Autodesk Fusion 360 part; units mm, degrees
(part 4 of 8)
  spline S46 degree 5 poles (-31.9025, -58.9172) (-31.888, -58.9061) (-31.859, -58.884) (-31.8155, -58.8507) (-31.7578, -58.8063) (-31.6858, -58.7505) (-31.6141, -58.6945) (-31.5426, -58.6384) (-31.4714, -58.582) (-31.4004, -58.5254) (-31.3297, -58.4686) (-31.2593, -58.4117) (-31.1891, -58.3545) (-31.1191, -58.2971) (-31.0494, -58.2395) (-30.98, -58.1817) (-30.9109, -58.1237) (-30.842, -58.0655) (-30.7734, -58.0071) (-30.705, -57.9485) (-30.637, -57.8897) (-30.5692, -57.8306) (-30.5017, -57.7714) (-30.4345, -57.7119) (-30.3675, -57.6522) (-30.3009, -57.5923) (-30.2346, -57.5322) (-30.1685, -57.4719) (-30.1028, -57.4113) (-30.0373, -57.3505) (-29.9722, -57.2895) (-29.9073, -57.2283) (-29.8428, -57.1669) (-29.7786, -57.1052) (-29.7147, -57.0433) (-29.6512, -56.9812) (-29.588, -56.9188) (-29.5251, -56.8563) (-29.4626, -56.7934) (-29.4004, -56.7304) (-29.3385, -56.6671) (-29.277, -56.6035) (-29.2159, -56.5397) (-29.1551, -56.4757) (-29.0947, -56.4114) (-29.0347, -56.3469) (-28.9751, -56.2821) (-28.9158, -56.217) (-28.857, -56.1517) (-28.7986, -56.0861) (-28.7406, -56.0202) (-28.683, -55.9541) (-28.6369, -55.9004) (-28.6023, -55.8599) (-28.5792, -55.8327) (-28.5675, -55.8188) (-28.567, -55.8182) knots -1 -1 -1 -1 -1 -1 -0.985714 -0.971429 -0.957143 -0.942857 -0.928571 -0.914286 -0.9 -0.885714 -0.871429 -0.857143 -0.842857 -0.828571 -0.814286 -0.8 -0.785714 -0.771429 -0.757143 -0.742857 -0.728571 -0.714286 -0.7 -0.685714 -0.671429 -0.657143 -0.642857 -0.628571 -0.614286 -0.6 -0.585714 -0.571429 -0.557143 -0.542857 -0.528571 -0.514286 -0.5 -0.485714 -0.471429 -0.457143 -0.442857 -0.428571 -0.414286 -0.4 -0.385714 -0.371429 -0.357143 -0.342857 -0.328571 -0.314286 -0.3 -0.285714 -0.271429 -0.270845 -0.270845 -0.270845 -0.270845 -0.270845 -0.270845
  spline S47 degree 3 poles (-28.3236, -55.7689) (-28.3469, -55.7571) (-28.3722, -55.75) (-28.4241, -55.7458) (-28.4502, -55.7488) (-28.4928, -55.7624) (-28.5098, -55.7706) (-28.5409, -55.7914) (-28.5549, -55.8039) (-28.567, -55.8182) knots 0 0 0 0 0.007813 0.007813 0.015626 0.015626 0.021241 0.021241 0.026855 0.026855 0.026855 0.026855
  arc A24 (-28.3236, -55.7689) -> (-27.1157, -56.3661) centre (0, 0) ccw
  spline S48 degree 3 poles (-27.0071, -56.5894) (-27.0015, -56.564) (-27.0009, -56.5377) (-27.0098, -56.4864) (-27.0193, -56.4619) (-27.0431, -56.424) (-27.0553, -56.4096) (-27.0832, -56.3847) (-27.0988, -56.3743) (-27.1157, -56.3661) knots 0 0 0 0 0.007813 0.007813 0.015626 0.015626 0.021241 0.021241 0.026855 0.026855 0.026855 0.026855
  spline S49 degree 5 poles (-27.0071, -56.5894) (-27.0072, -56.5901) (-27.0112, -56.6079) (-27.0188, -56.6428) (-27.03, -56.6949) (-27.0446, -56.7641) (-27.0622, -56.85) (-27.0793, -56.9361) (-27.096, -57.0223) (-27.1122, -57.1087) (-27.1279, -57.1953) (-27.1432, -57.282) (-27.158, -57.3689) (-27.1724, -57.4559) (-27.1864, -57.5431) (-27.2, -57.6304) (-27.2131, -57.7178) (-27.2259, -57.8054) (-27.2382, -57.8931) (-27.2502, -57.981) (-27.2617, -58.0689) (-27.2729, -58.157) (-27.2837, -58.2452) (-27.2941, -58.3336) (-27.3041, -58.422) (-27.3137, -58.5106) (-27.323, -58.5993) (-27.3319, -58.6881) (-27.3405, -58.777) (-27.3487, -58.866) (-27.3565, -58.9551) (-27.364, -59.0443) (-27.3711, -59.1336) (-27.3779, -59.223) (-27.3843, -59.3126) (-27.3904, -59.4022) (-27.3962, -59.4919) (-27.4016, -59.5817) (-27.4067, -59.6716) (-27.4115, -59.7616) (-27.4159, -59.8516) (-27.42, -59.9418) (-27.4238, -60.032) (-27.4272, -60.1224) (-27.4303, -60.2128) (-27.4331, -60.3033) (-27.4356, -60.3939) (-27.4378, -60.4845) (-27.4397, -60.5753) (-27.4412, -60.6661) (-27.4425, -60.757) (-27.4434, -60.8479) (-27.444, -60.939) (-27.4443, -61.0119) (-27.4443, -61.0666) (-27.4443, -61.103) (-27.4443, -61.1213) knots 0.270845 0.270845 0.270845 0.270845 0.270845 0.270845 0.271429 0.285714 0.3 0.314286 0.328571 0.342857 0.357143 0.371429 0.385714 0.4 0.414286 0.428571 0.442857 0.457143 0.471429 0.485714 0.5 0.514286 0.528571 0.542857 0.557143 0.571429 0.585714 0.6 0.614286 0.628571 0.642857 0.657143 0.671429 0.685714 0.7 0.714286 0.728571 0.742857 0.757143 0.771429 0.785714 0.8 0.814286 0.828571 0.842857 0.857143 0.871429 0.885714 0.9 0.914286 0.928571 0.942857 0.957143 0.971429 0.985714 1 1 1 1 1 1
  arc A25 (-27.4443, -61.1213) -> (-26.0672, -61.7211) centre (0, 0) ccw
  spline S50 degree 5 poles (-26.0672, -61.7211) (-26.0538, -61.7087) (-26.0271, -61.6839) (-25.9871, -61.6466) (-25.9339, -61.5968) (-25.8676, -61.5343) (-25.8017, -61.4717) (-25.736, -61.4089) (-25.6705, -61.3459) (-25.6053, -61.2828) (-25.5404, -61.2194) (-25.4758, -61.1559) (-25.4114, -61.0922) (-25.3474, -61.0284) (-25.2836, -60.9643) (-25.2201, -60.9001) (-25.1568, -60.8357) (-25.0939, -60.7711) (-25.0312, -60.7064) (-24.9689, -60.6414) (-24.9068, -60.5763) (-24.845, -60.511) (-24.7836, -60.4455) (-24.7224, -60.3798) (-24.6615, -60.314) (-24.601, -60.2479) (-24.5408, -60.1817) (-24.4808, -60.1152) (-24.4212, -60.0486) (-24.362, -59.9818) (-24.303, -59.9148) (-24.2444, -59.8476) (-24.1861, -59.7803) (-24.1282, -59.7127) (-24.0706, -59.6449) (-24.0133, -59.5769) (-23.9564, -59.5088) (-23.8998, -59.4404) (-23.8437, -59.3718) (-23.7878, -59.3031) (-23.7324, -59.2341) (-23.6773, -59.1649) (-23.6226, -59.0955) (-23.5683, -59.0259) (-23.5144, -58.9561) (-23.4609, -58.8861) (-23.4078, -58.8158) (-23.3551, -58.7453) (-23.3029, -58.6747) (-23.2511, -58.6037) (-23.1997, -58.5326) (-23.1488, -58.4612) (-23.108, -58.4033) (-23.0775, -58.3597) (-23.0572, -58.3303) (-23.0468, -58.3153) (-23.0464, -58.3147) knots -1 -1 -1 -1 -1 -1 -0.985714 -0.971429 -0.957143 -0.942857 -0.928571 -0.914286 -0.9 -0.885714 -0.871429 -0.857143 -0.842857 -0.828571 -0.814286 -0.8 -0.785714 -0.771429 -0.757143 -0.742857 -0.728571 -0.714286 -0.7 -0.685714 -0.671429 -0.657143 -0.642857 -0.628571 -0.614286 -0.6 -0.585714 -0.571429 -0.557143 -0.542857 -0.528571 -0.514286 -0.5 -0.485714 -0.471429 -0.457143 -0.442857 -0.428571 -0.414286 -0.4 -0.385714 -0.371429 -0.357143 -0.342857 -0.328571 -0.314286 -0.3 -0.285714 -0.271429 -0.270845 -0.270845 -0.270845 -0.270845 -0.270845 -0.270845
  spline S51 degree 3 poles (-22.8089, -58.2422) (-22.8332, -58.2327) (-22.8591, -58.228) (-22.9111, -58.2289) (-22.9368, -58.2344) (-22.978, -58.252) (-22.994, -58.2618) (-23.023, -58.2855) (-23.0358, -58.2993) (-23.0464, -58.3147) knots 0 0 0 0 0.007813 0.007813 0.015626 0.015626 0.021241 0.021241 0.026855 0.026855 0.026855 0.026855
  arc A26 (-22.8089, -58.2422) -> (-21.549, -58.72) centre (0, 0) ccw
  spline S52 degree 3 poles (-21.4193, -58.9318) (-21.4162, -58.9059) (-21.4182, -58.8797) (-21.432, -58.8295) (-21.4438, -58.806) (-21.4712, -58.7706) (-21.4846, -58.7575) (-21.5148, -58.7354) (-21.5314, -58.7265) (-21.549, -58.72) knots 0 0 0 0 0.007813 0.007813 0.015626 0.015626 0.021241 0.021241 0.026855 0.026855 0.026855 0.026855
  spline S53 degree 5 poles (-21.4193, -58.9318) (-21.4194, -58.9325) (-21.4216, -58.9506) (-21.4258, -58.9861) (-21.432, -59.039) (-21.4398, -59.1093) (-21.449, -59.1965) (-21.4578, -59.2838) (-21.466, -59.3713) (-21.4738, -59.4588) (-21.4811, -59.5465) (-21.488, -59.6343) (-21.4943, -59.7222) (-21.5003, -59.8102) (-21.5058, -59.8983) (-21.5109, -59.9865) (-21.5155, -60.0748) (-21.5198, -60.1632) (-21.5236, -60.2517) (-21.527, -60.3403) (-21.53, -60.429) (-21.5326, -60.5177) (-21.5348, -60.6066) (-21.5366, -60.6955) (-21.5381, -60.7845) (-21.5391, -60.8736) (-21.5398, -60.9628) (-21.5401, -61.052) (-21.54, -61.1413) (-21.5396, -61.2307) (-21.5388, -61.3202) (-21.5376, -61.4097) (-21.5361, -61.4993) (-21.5342, -61.5889) (-21.532, -61.6786) (-21.5294, -61.7684) (-21.5265, -61.8583) (-21.5232, -61.9482) (-21.5196, -62.0381) (-21.5157, -62.1282) (-21.5114, -62.2182) (-21.5068, -62.3084) (-21.5018, -62.3986) (-21.4965, -62.4888) (-21.4909, -62.5791) (-21.485, -62.6695) (-21.4787, -62.7599) (-21.4721, -62.8503) (-21.4652, -62.9408) (-21.458, -63.0313) (-21.4505, -63.1219) (-21.4426, -63.2125) (-21.4344, -63.3032) (-21.4277, -63.3758) (-21.4224, -63.4302) (-21.4189, -63.4665) (-21.4171, -63.4847) knots 0.270845 0.270845 0.270845 0.270845 0.270845 0.270845 0.271429 0.285714 0.3 0.314286 0.328571 0.342857 0.357143 0.371429 0.385714 0.4 0.414286 0.428571 0.442857 0.457143 0.471429 0.485714 0.5 0.514286 0.528571 0.542857 0.557143 0.571429 0.585714 0.6 0.614286 0.628571 0.642857 0.657143 0.671429 0.685714 0.7 0.714286 0.728571 0.742857 0.757143 0.771429 0.785714 0.8 0.814286 0.828571 0.842857 0.857143 0.871429 0.885714 0.9 0.914286 0.928571 0.942857 0.957143 0.971429 0.985714 1 1 1 1 1 1
  arc A27 (-21.4171, -63.4847) -> (-19.9886, -63.9489) centre (0, 0) ccw
  spline S54 degree 5 poles (-19.9886, -63.9489) (-19.9765, -63.9352) (-19.9522, -63.9079) (-19.916, -63.867) (-19.8679, -63.8122) (-19.808, -63.7437) (-19.7483, -63.675) (-19.689, -63.6061) (-19.6299, -63.5371) (-19.5712, -63.468) (-19.5127, -63.3987) (-19.4545, -63.3292) (-19.3966, -63.2596) (-19.3389, -63.1899) (-19.2816, -63.12) (-19.2246, -63.0499) (-19.1679, -62.9797) (-19.1115, -62.9093) (-19.0554, -62.8388) (-18.9996, -62.7682) (-18.9441, -62.6974) (-18.8889, -62.6264) (-18.834, -62.5553) (-18.7795, -62.484) (-18.7253, -62.4126) (-18.6714, -62.341) (-18.6178, -62.2692) (-18.5646, -62.1973) (-18.5117, -62.1253) (-18.4591, -62.0531) (-18.4069, -61.9807) (-18.3551, -61.9082) (-18.3036, -61.8355) (-18.2524, -61.7626) (-18.2016, -61.6896) (-18.1512, -61.6164) (-18.1011, -61.5431) (-18.0514, -61.4696) (-18.0021, -61.3959) (-17.9532, -61.3221) (-17.9047, -61.2481) (-17.8565, -61.1739) (-17.8088, -61.0995) (-17.7615, -61.025) (-17.7145, -60.9503) (-17.6681, -60.8755) (-17.622, -60.8004) (-17.5764, -60.7252) (-17.5312, -60.6498) (-17.4865, -60.5742) (-17.4422, -60.4984) (-17.3984, -60.4225) (-17.3634, -60.3609) (-17.3373, -60.3145) (-17.3198, -60.2833) (-17.311, -60.2674) (-17.3106, -60.2668) knots -1 -1 -1 -1 -1 -1 -0.985714 -0.971429 -0.957143 -0.942857 -0.928571 -0.914286 -0.9 -0.885714 -0.871429 -0.857143 -0.842857 -0.828571 -0.814286 -0.8 -0.785714 -0.771429 -0.757143 -0.742857 -0.728571 -0.714286 -0.7 -0.685714 -0.671429 -0.657143 -0.642857 -0.628571 -0.614286 -0.6 -0.585714 -0.571429 -0.557143 -0.542857 -0.528571 -0.514286 -0.5 -0.485714 -0.471429 -0.457143 -0.442857 -0.428571 -0.414286 -0.4 -0.385714 -0.371429 -0.357143 -0.342857 -0.328571 -0.314286 -0.3 -0.285714 -0.271429 -0.270845 -0.270845 -0.270845 -0.270845 -0.270845 -0.270845
  spline S55 degree 3 poles (-17.0813, -60.1717) (-17.1063, -60.1646) (-17.1325, -60.1624) (-17.1843, -60.1683) (-17.2093, -60.1763) (-17.2486, -60.1978) (-17.2636, -60.2091) (-17.2902, -60.2355) (-17.3015, -60.2505) (-17.3106, -60.2668) knots 0 0 0 0 0.007813 0.007813 0.015626 0.015626 0.021241 0.021241 0.026855 0.026855 0.026855 0.026855
  arc A28 (-17.0813, -60.1717) -> (-15.7811, -60.5257) centre (0, 0) ccw
  spline S56 degree 3 poles (-15.6316, -60.724) (-15.631, -60.6979) (-15.6355, -60.672) (-15.6541, -60.6234) (-15.6681, -60.6011) (-15.6988, -60.5685) (-15.7134, -60.5568) (-15.7456, -60.5377) (-15.763, -60.5304) (-15.7811, -60.5257) knots 0 0 0 0 0.007813 0.007813 0.015626 0.015626 0.021241 0.021241 0.026855 0.026855 0.026855 0.026855
  spline S57 degree 5 poles (-15.6316, -60.724) (-15.6316, -60.7247) (-15.6321, -60.7429) (-15.6328, -60.7786) (-15.6338, -60.8318) (-15.6349, -60.9026) (-15.6356, -60.9903) (-15.6359, -61.0781) (-15.6357, -61.1659) (-15.6349, -61.2538) (-15.6338, -61.3418) (-15.6321, -61.4298) (-15.63, -61.5179) (-15.6274, -61.6061) (-15.6244, -61.6943) (-15.6209, -61.7826) (-15.617, -61.8709) (-15.6127, -61.9593) (-15.608, -62.0478) (-15.6028, -62.1363) (-15.5973, -62.2248) (-15.5913, -62.3134) (-15.5849, -62.4021) (-15.5781, -62.4908) (-15.571, -62.5795) (-15.5634, -62.6683) (-15.5555, -62.7571) (-15.5472, -62.8459) (-15.5385, -62.9348) (-15.5294, -63.0237) (-15.52, -63.1127) (-15.5102, -63.2017) (-15.5, -63.2907) (-15.4895, -63.3798) (-15.4786, -63.4688) (-15.4674, -63.558) (-15.4558, -63.6471) (-15.4439, -63.7363) (-15.4316, -63.8255) (-15.419, -63.9147) (-15.406, -64.0039) (-15.3927, -64.0932) (-15.3791, -64.1825) (-15.3651, -64.2718) (-15.3508, -64.3611) (-15.3362, -64.4505) (-15.3212, -64.5399) (-15.306, -64.6292) (-15.2903, -64.7187) (-15.2744, -64.8081) (-15.2582, -64.8975) (-15.2416, -64.987) (-15.2247, -65.0764) (-15.211, -65.148) (-15.2005, -65.2017) (-15.1935, -65.2375) (-15.19, -65.2554) knots 0.270845 0.270845 0.270845 0.270845 0.270845 0.270845 0.271429 0.285714 0.3 0.314286 0.328571 0.342857 0.357143 0.371429 0.385714 0.4 0.414286 0.428571 0.442857 0.457143 0.471429 0.485714 0.5 0.514286 0.528571 0.542857 0.557143 0.571429 0.585714 0.6 0.614286 0.628571 0.642857 0.657143 0.671429 0.685714 0.7 0.714286 0.728571 0.742857 0.757143 0.771429 0.785714 0.8 0.814286 0.828571 0.842857 0.857143 0.871429 0.885714 0.9 0.914286 0.928571 0.942857 0.957143 0.971429 0.985714 1 1 1 1 1 1
  arc A29 (-15.19, -65.2554) -> (-13.7233, -65.5795) centre (0, 0) ccw
  spline S58 degree 5 poles (-13.7233, -65.5795) (-13.7126, -65.5648) (-13.6911, -65.5353) (-13.659, -65.491) (-13.6163, -65.4319) (-13.5633, -65.3578) (-13.5106, -65.2837) (-13.4582, -65.2094) (-13.4061, -65.1351) (-13.3543, -65.0606) (-13.3027, -64.9859) (-13.2515, -64.9112) (-13.2006, -64.8363) (-13.15, -64.7613) (-13.0997, -64.6862) (-13.0497, -64.611) (-13, -64.5356) (-12.9506, -64.4602) (-12.9016, -64.3846) (-12.8529, -64.3089) (-12.8045, -64.233) (-12.7564, -64.1571) (-12.7087, -64.081) (-12.6612, -64.0048) (-12.6142, -63.9285) (-12.5674, -63.852) (-12.5211, -63.7754) (-12.475, -63.6987) (-12.4293, -63.6219) (-12.384, -63.545) (-12.339, -63.4679) (-12.2944, -63.3907) (-12.2501, -63.3134) (-12.2063, -63.2359) (-12.1627, -63.1583) (-12.1196, -63.0806) (-12.0769, -63.0028) (-12.0345, -62.9248) (-11.9925, -62.8468) (-11.951, -62.7685) (-11.9098, -62.6902) (-11.869, -62.6117) (-11.8287, -62.5331) (-11.7888, -62.4544) (-11.7493, -62.3755) (-11.7102, -62.2965) (-11.6716, -62.2174) (-11.6335, -62.1381) (-11.5958, -62.0587) (-11.5586, -61.9791) (-11.5218, -61.8994) (-11.4856, -61.8196) (-11.4567, -61.7549) (-11.4351, -61.7062) (-11.4208, -61.6735) (-11.4135, -61.6568) (-11.4132, -61.6562) knots -1 -1 -1 -1 -1 -1 -0.985714 -0.971429 -0.957143 -0.942857 -0.928571 -0.914286 -0.9 -0.885714 -0.871429 -0.857143 -0.842857 -0.828571 -0.814286 -0.8 -0.785714 -0.771429 -0.757143 -0.742857 -0.728571 -0.714286 -0.7 -0.685714 -0.671429 -0.657143 -0.642857 -0.628571 -0.614286 -0.6 -0.585714 -0.571429 -0.557143 -0.542857 -0.528571 -0.514286 -0.5 -0.485714 -0.471429 -0.457143 -0.442857 -0.428571 -0.414286 -0.4 -0.385714 -0.371429 -0.357143 -0.342857 -0.328571 -0.314286 -0.3 -0.285714 -0.271429 -0.270845 -0.270845 -0.270845 -0.270845 -0.270845 -0.270845
  spline S59 degree 3 poles (-11.1941, -61.5394) (-11.2197, -61.5347) (-11.246, -61.5351) (-11.297, -61.5459) (-11.3212, -61.5563) (-11.3581, -61.5815) (-11.372, -61.5942) (-11.3959, -61.623) (-11.4058, -61.639) (-11.4132, -61.6562) knots 0 0 0 0 0.007813 0.007813 0.015626 0.015626 0.021241 0.021241 0.026855 0.026855 0.026855 0.026855
  arc A30 (-11.1941, -61.5394) -> (-9.8659, -61.7662) centre (0, 0) ccw
  spline S60 degree 3 poles (-9.6979, -61.9491) (-9.6998, -61.9232) (-9.7068, -61.8978) (-9.73, -61.8512) (-9.7461, -61.8304) (-9.7798, -61.8009) (-9.7955, -61.7906) (-9.8294, -61.7747) (-9.8474, -61.7692) (-9.8659, -61.7662) knots 0 0 0 0 0.007813 0.007813 0.015626 0.015626 0.021241 0.021241 0.026855 0.026855 0.026855 0.026855
  spline S61 degree 5 poles (-9.6979, -61.9491) (-9.6979, -61.9499) (-9.6965, -61.968) (-9.6939, -62.0036) (-9.6897, -62.0567) (-9.6839, -62.1273) (-9.6762, -62.2146) (-9.668, -62.302) (-9.6593, -62.3894) (-9.6501, -62.4768) (-9.6404, -62.5643) (-9.6303, -62.6517) (-9.6197, -62.7392) (-9.6086, -62.8267) (-9.5971, -62.9143) (-9.5851, -63.0018) (-9.5727, -63.0894) (-9.5599, -63.1769) (-9.5466, -63.2645) (-9.533, -63.3521) (-9.5189, -63.4397) (-9.5044, -63.5273) (-9.4895, -63.6149) (-9.4742, -63.7025) (-9.4585, -63.7902) (-9.4424, -63.8778) (-9.426, -63.9654) (-9.4091, -64.053) (-9.3919, -64.1407) (-9.3743, -64.2283) (-9.3563, -64.3159) (-9.338, -64.4036) (-9.3193, -64.4912) (-9.3002, -64.5788) (-9.2808, -64.6665) (-9.261, -64.7541) (-9.2408, -64.8417) (-9.2204, -64.9293) (-9.1995, -65.0169) (-9.1784, -65.1045) (-9.1568, -65.192) (-9.135, -65.2796) (-9.1128, -65.3672) (-9.0903, -65.4547) (-9.0674, -65.5422) (-9.0442, -65.6298) (-9.0207, -65.7173) (-8.9969, -65.8048) (-8.9727, -65.8923) (-8.9482, -65.9797) (-8.9234, -66.0672) (-8.8983, -66.1546) (-8.8729, -66.242) (-8.8523, -66.3119) (-8.8367, -66.3644) (-8.8262, -66.3993) (-8.821, -66.4168) knots 0.270845 0.270845 0.270845 0.270845 0.270845 0.270845 0.271429 0.285714 0.3 0.314286 0.328571 0.342857 0.357143 0.371429 0.385714 0.4 0.414286 0.428571 0.442857 0.457143 0.471429 0.485714 0.5 0.514286 0.528571 0.542857 0.557143 0.571429 0.585714 0.6 0.614286 0.628571 0.642857 0.657143 0.671429 0.685714 0.7 0.714286 0.728571 0.742857 0.757143 0.771429 0.785714 0.8 0.814286 0.828571 0.842857 0.857143 0.871429 0.885714 0.9 0.914286 0.928571 0.942857 0.957143 0.971429 0.985714 1 1 1 1 1 1
  arc A31 (-8.821, -66.4168) -> (-7.3299, -66.5978) centre (0, 0) ccw
  spline S62 degree 5 poles (-7.3299, -66.5978) (-7.3206, -66.5821) (-7.3021, -66.5507) (-7.2744, -66.5035) (-7.2377, -66.4406) (-7.1921, -66.3618) (-7.1468, -66.2829) (-7.1018, -66.2039) (-7.0571, -66.1249) (-7.0127, -66.0457) (-6.9686, -65.9665) (-6.9248, -65.8871) (-6.8813, -65.8077) (-6.8382, -65.7282) (-6.7954, -65.6485) (-6.7529, -65.5688) (-6.7107, -65.4891) (-6.6689, -65.4092) (-6.6273, -65.3292) (-6.5862, -65.2491) (-6.5453, -65.169) (-6.5048, -65.0887) (-6.4646, -65.0084) (-6.4248, -64.928) (-6.3853, -64.8475) (-6.3462, -64.7668) (-6.3074, -64.6862) (-6.269, -64.6054) (-6.2309, -64.5245) (-6.1932, -64.4435) (-6.1559, -64.3625) (-6.1189, -64.2813) (-6.0823, -64.2001) (-6.0461, -64.1188) (-6.0103, -64.0374) (-5.9749, -63.9559) (-5.9398, -63.8743) (-5.9052, -63.7926) (-5.871, -63.7108) (-5.8371, -63.6289) (-5.8037, -63.547) (-5.7707, -63.465) (-5.7382, -63.3828) (-5.706, -63.3006) (-5.6743, -63.2183) (-5.6431, -63.1359) (-5.6123, -63.0534) (-5.582, -62.9708) (-5.5521, -62.8881) (-5.5228, -62.8053) (-5.4939, -62.7225) (-5.4655, -62.6395) (-5.443, -62.5724) (-5.4262, -62.5218) (-5.4151, -62.4879) (-5.4095, -62.4706) (-5.4093, -62.4699) knots -1 -1 -1 -1 -1 -1 -0.985714 -0.971429 -0.957143 -0.942857 -0.928571 -0.914286 -0.9 -0.885714 -0.871429 -0.857143 -0.842857 -0.828571 -0.814286 -0.8 -0.785714 -0.771429 -0.757143 -0.742857 -0.728571 -0.714286 -0.7 -0.685714 -0.671429 -0.657143 -0.642857 -0.628571 -0.614286 -0.6 -0.585714 -0.571429 -0.557143 -0.542857 -0.528571 -0.514286 -0.5 -0.485714 -0.471429 -0.457143 -0.442857 -0.428571 -0.414286 -0.4 -0.385714 -0.371429 -0.357143 -0.342857 -0.328571 -0.314286 -0.3 -0.285714 -0.271429 -0.270845 -0.270845 -0.270845 -0.270845 -0.270845 -0.270845
  spline S63 degree 3 poles (-5.2025, -62.3325) (-5.2284, -62.3303) (-5.2545, -62.3332) (-5.3042, -62.3489) (-5.3273, -62.3616) (-5.3616, -62.3902) (-5.3742, -62.4042) (-5.3952, -62.4352) (-5.4035, -62.4521) (-5.4093, -62.4699) knots 0 0 0 0 0.007813 0.007813 0.015626 0.015626 0.021241 0.021241 0.026855 0.026855 0.026855 0.026855
  arc A32 (-5.2025, -62.3325) -> (-3.8585, -62.4301) centre (0, 0) ccw
  spline S64 degree 3 poles (-3.6737, -62.5959) (-3.6781, -62.5703) (-3.6875, -62.5457) (-3.7151, -62.5015) (-3.7331, -62.4824) (-3.7695, -62.4563) (-3.7861, -62.4476) (-3.8214, -62.435) (-3.8398, -62.4312) (-3.8585, -62.4301) knots 0 0 0 0 0.007813 0.007813 0.015626 0.015626 0.021241 0.021241 0.026855 0.026855 0.026855 0.026855
  spline S65 degree 5 poles (-3.6737, -62.5959) (-3.6736, -62.5966) (-3.6705, -62.6146) (-3.6644, -62.6498) (-3.6552, -62.7022) (-3.6426, -62.7719) (-3.6265, -62.8581) (-3.6099, -62.9443) (-3.5928, -63.0304) (-3.5752, -63.1165) (-3.5571, -63.2026) (-3.5386, -63.2887) (-3.5196, -63.3748) (-3.5001, -63.4608) (-3.4802, -63.5468) (-3.4598, -63.6328) (-3.439, -63.7187) (-3.4178, -63.8047) (-3.3962, -63.8905) (-3.3741, -63.9764) (-3.3516, -64.0622) (-3.3287, -64.148) (-3.3055, -64.2338) (-3.2818, -64.3195) (-3.2577, -64.4052) (-3.2332, -64.4909) (-3.2084, -64.5765) (-3.1832, -64.6621) (-3.1576, -64.7477) (-3.1316, -64.8332) (-3.1052, -64.9187) (-3.0785, -65.0042) (-3.0515, -65.0896) (-3.024, -65.175) (-2.9962, -65.2603) (-2.9681, -65.3456) (-2.9396, -65.4308) (-2.9107, -65.5161) (-2.8816, -65.6012) (-2.852, -65.6864) (-2.8222, -65.7715) (-2.792, -65.8565) (-2.7614, -65.9415) (-2.7306, -66.0265) (-2.6994, -66.1114) (-2.6678, -66.1963) (-2.636, -66.2811) (-2.6038, -66.3659) (-2.5713, -66.4506) (-2.5385, -66.5353) (-2.5054, -66.62) (-2.4719, -66.7046) (-2.4382, -66.7891) (-2.4109, -66.8567) (-2.3904, -66.9074) (-2.3766, -66.9412) (-2.3697, -66.9581) knots 0.270845 0.270845 0.270845 0.270845 0.270845 0.270845 0.271429 0.285714 0.3 0.314286 0.328571 0.342857 0.357143 0.371429 0.385714 0.4 0.414286 0.428571 0.442857 0.457143 0.471429 0.485714 0.5 0.514286 0.528571 0.542857 0.557143 0.571429 0.585714 0.6 0.614286 0.628571 0.642857 0.657143 0.671429 0.685714 0.7 0.714286 0.728571 0.742857 0.757143 0.771429 0.785714 0.8 0.814286 0.828571 0.842857 0.857143 0.871429 0.885714 0.9 0.914286 0.928571 0.942857 0.957143 0.971429 0.985714 1 1 1 1 1 1
  arc A33 (-2.3697, -66.9581) -> (-0.8681, -66.9944) centre (0, 0) ccw
  spline S66 degree 5 poles (-0.8681, -66.9944) (-0.8604, -66.9778) (-0.845, -66.9448) (-0.822, -66.8951) (-0.7915, -66.8289) (-0.7537, -66.7461) (-0.7162, -66.6632) (-0.679, -66.5803) (-0.6421, -66.4973) (-0.6056, -66.4142) (-0.5694, -66.3311) (-0.5335, -66.2479) (-0.4979, -66.1646) (-0.4626, -66.0813) (-0.4277, -65.9979) (-0.3931, -65.9145) (-0.3588, -65.831) (-0.3248, -65.7475) (-0.2912, -65.6638) (-0.258, -65.5802) (-0.225, -65.4965) (-0.1925, -65.4127) (-0.1602, -65.3288) (-0.1283, -65.2449) (-0.0968, -65.161) (-0.0656, -65.077) (-0.0348, -64.9929) (-0.0044, -64.9088) (0.0257, -64.8246) (0.0554, -64.7404) (0.0847, -64.6561) (0.1137, -64.5718) (0.1423, -64.4874) (0.1705, -64.403) (0.1983, -64.3185) (0.2257, -64.2339) (0.2526, -64.1494) (0.2792, -64.0647) (0.3054, -63.98) (0.3312, -63.8953) (0.3565, -63.8105) (0.3815, -63.7256) (0.4059, -63.6407) (0.43, -63.5558) (0.4536, -63.4708) (0.4767, -63.3858) (0.4994, -63.3007) (0.5216, -63.2156) (0.5434, -63.1304) (0.5646, -63.0452) (0.5853, -62.9599) (0.6056, -62.8746) (0.6215, -62.8056) (0.6333, -62.7537) (0.6411, -62.7188) (0.645, -62.701) (0.6452, -62.7003) knots -1 -1 -1 -1 -1 -1 -0.985714 -0.971429 -0.957143 -0.942857 -0.928571 -0.914286 -0.9 -0.885714 -0.871429 -0.857143 -0.842857 -0.828571 -0.814286 -0.8 -0.785714 -0.771429 -0.757143 -0.742857 -0.728571 -0.714286 -0.7 -0.685714 -0.671429 -0.657143 -0.642857 -0.628571 -0.614286 -0.6 -0.585714 -0.571429 -0.557143 -0.542857 -0.528571 -0.514286 -0.5 -0.485714 -0.471429 -0.457143 -0.442857 -0.428571 -0.414286 -0.4 -0.385714 -0.371429 -0.357143 -0.342857 -0.328571 -0.314286 -0.3 -0.285714 -0.271429 -0.270845 -0.270845 -0.270845 -0.270845 -0.270845 -0.270845
  spline S67 degree 3 poles (0.8378, -62.5436) (0.8117, -62.5439) (0.786, -62.5494) (0.7381, -62.5698) (0.7164, -62.5846) (0.6849, -62.6164) (0.6737, -62.6315) (0.6558, -62.6644) (0.6492, -62.682) (0.6452, -62.7003) knots 0 0 0 0 0.007813 0.007813 0.015626 0.015626 0.021241 0.021241 0.026855 0.026855 0.026855 0.026855
  arc A34 (0.8378, -62.5436) -> (2.1849, -62.511) centre (0, 0) ccw
  spline S68 degree 3 poles (2.3848, -62.6583) (2.378, -62.6331) (2.3663, -62.6096) (2.3345, -62.5683) (2.3148, -62.551) (2.276, -62.5285) (2.2586, -62.5214) (2.2223, -62.5123) (2.2036, -62.5104) (2.1849, -62.511) knots 0 0 0 0 0.007813 0.007813 0.015626 0.015626 0.021241 0.021241 0.026855 0.026855 0.026855 0.026855
  spline S69 degree 5 poles (2.3848, -62.6583) (2.385, -62.659) (2.3898, -62.6765) (2.3993, -62.711) (2.4135, -62.7623) (2.4328, -62.8304) (2.4571, -62.9146) (2.482, -62.9988) (2.5073, -63.0829) (2.5331, -63.1669) (2.5594, -63.2509) (2.5862, -63.3348) (2.6134, -63.4186) (2.6411, -63.5024) (2.6692, -63.586) (2.6978, -63.6696) (2.7268, -63.7532) (2.7562, -63.8367) (2.786, -63.9201) (2.8163, -64.0034) (2.8469, -64.0866) (2.878, -64.1698) (2.9094, -64.253) (2.9413, -64.336) (2.9735, -64.419) (3.0061, -64.5019) (3.0391, -64.5847) (3.0725, -64.6675) (3.1062, -64.7502) (3.1403, -64.8328) (3.1748, -64.9153) (3.2097, -64.9978) (3.2448, -65.0802) (3.2804, -65.1626) (3.3163, -65.2448) (3.3525, -65.327) (3.3891, -65.4091) (3.4261, -65.4911) (3.4633, -65.5731) (3.5009, -65.655) (3.5389, -65.7368) (3.5771, -65.8185) (3.6157, -65.9002) (3.6547, -65.9818) (3.6939, -66.0633) (3.7335, -66.1447) (3.7734, -66.2261) (3.8136, -66.3074) (3.8541, -66.3886) (3.8949, -66.4697) (3.9361, -66.5508) (3.9775, -66.6318) (4.0193, -66.7127) (4.0529, -66.7773) (4.0783, -66.8258) (4.0953, -66.8581) (4.1038, -66.8742) knots 0.270845 0.270845 0.270845 0.270845 0.270845 0.270845 0.271429 0.285714 0.3 0.314286 0.328571 0.342857 0.357143 0.371429 0.385714 0.4 0.414286 0.428571 0.442857 0.457143 0.471429 0.485714 0.5 0.514286 0.528571 0.542857 0.557143 0.571429 0.585714 0.6 0.614286 0.628571 0.642857 0.657143 0.671429 0.685714 0.7 0.714286 0.728571 0.742857 0.757143 0.771429 0.785714 0.8 0.814286 0.828571 0.842857 0.857143 0.871429 0.885714 0.9 0.914286 0.928571 0.942857 0.957143 0.971429 0.985714 1 1 1 1 1 1
  arc A35 (4.1038, -66.8742) -> (5.6019, -66.7654) centre (0, 0) ccw
  spline S70 degree 5 poles (5.6019, -66.7654) (5.608, -66.7482) (5.6201, -66.7138) (5.6382, -66.6622) (5.6621, -66.5933) (5.6918, -66.5073) (5.7211, -66.4211) (5.7501, -66.335) (5.7788, -66.2488) (5.8071, -66.1626) (5.8352, -66.0764) (5.8629, -65.9901) (5.8903, -65.9038) (5.9173, -65.8175) (5.9441, -65.7311) (5.9704, -65.6447) (5.9965, -65.5583) (6.0222, -65.4719) (6.0476, -65.3854) (6.0726, -65.2989) (6.0973, -65.2124) (6.1217, -65.1259) (6.1457, -65.0393) (6.1693, -64.9527) (6.1926, -64.8661) (6.2155, -64.7795) (6.2381, -64.6929) (6.2602, -64.6062) (6.2821, -64.5195) (6.3035, -64.4328) (6.3246, -64.3461) (6.3452, -64.2594) (6.3655, -64.1726) (6.3854, -64.0859) (6.405, -63.9991) (6.4241, -63.9123) (6.4428, -63.8255) (6.4611, -63.7387) (6.479, -63.6519) (6.4964, -63.565) (6.5135, -63.4782) (6.5301, -63.3913) (6.5463, -63.3045) (6.562, -63.2176) (6.5773, -63.1307) (6.5921, -63.0438) (6.6065, -62.957) (6.6204, -62.8701) (6.6338, -62.7832) (6.6467, -62.6963) (6.6591, -62.6095) (6.671, -62.5226) (6.6803, -62.4524) (6.687, -62.3996) (6.6913, -62.3641) (6.6935, -62.346) (6.6936, -62.3453) knots -1 -1 -1 -1 -1 -1 -0.985714 -0.971429 -0.957143 -0.942857 -0.928571 -0.914286 -0.9 -0.885714 -0.871429 -0.857143 -0.842857 -0.828571 -0.814286 -0.8 -0.785714 -0.771429 -0.757143 -0.742857 -0.728571 -0.714286 -0.7 -0.685714 -0.671429 -0.657143 -0.642857 -0.628571 -0.614286 -0.6 -0.585714 -0.571429 -0.557143 -0.542857 -0.528571 -0.514286 -0.5 -0.485714 -0.471429 -0.457143 -0.442857 -0.428571 -0.414286 -0.4 -0.385714 -0.371429 -0.357143 -0.342857 -0.328571 -0.314286 -0.3 -0.285714 -0.271429 -0.270845 -0.270845 -0.270845 -0.270845 -0.270845 -0.270845
  spline S71 degree 3 poles (6.8702, -62.1708) (6.8443, -62.1736) (6.8192, -62.1815) (6.7735, -62.2065) (6.7533, -62.2233) (6.7251, -62.258) (6.7154, -62.2741) (6.7008, -62.3086) (6.6959, -62.3268) (6.6936, -62.3453) knots 0 0 0 0 0.007813 0.007813 0.015626 0.015626 0.021241 0.021241 0.026855 0.026855 0.026855 0.026855
  arc A36 (6.8702, -62.1708) -> (8.2079, -62.0083) centre (0, 0) ccw
  spline S72 degree 3 poles (8.4211, -62.1356) (8.4118, -62.1112) (8.3979, -62.0889) (8.3623, -62.0509) (8.341, -62.0356) (8.3003, -62.0169) (8.2823, -62.0116) (8.2452, -62.006) (8.2264, -62.0059) (8.2079, -62.0083) knots 0 0 0 0 0.007813 0.007813 0.015626 0.015626 0.021241 0.021241 0.026855 0.026855 0.026855 0.026855
  spline S73 degree 5 poles (8.4211, -62.1356) (8.4213, -62.1363) (8.4278, -62.1533) (8.4406, -62.1867) (8.4597, -62.2363) (8.4854, -62.3023) (8.5178, -62.3838) (8.5507, -62.4652) (8.584, -62.5464) (8.6178, -62.6276) (8.6521, -62.7086) (8.6868, -62.7895) (8.722, -62.8703) (8.7576, -62.951) (8.7937, -63.0316) (8.8302, -63.112) (8.8671, -63.1924) (8.9045, -63.2726) (8.9422, -63.3528) (8.9803, -63.4328) (9.0189, -63.5127) (9.0578, -63.5925) (9.0971, -63.6722) (9.1369, -63.7518) (9.177, -63.8313) (9.2174, -63.9106) (9.2583, -63.9899) (9.2995, -64.0691) (9.341, -64.1481) (9.3829, -64.227) (9.4252, -64.3059) (9.4679, -64.3846) (9.5108, -64.4632) (9.5542, -64.5417) (9.5978, -64.6202) (9.6418, -64.6985) (9.6862, -64.7766) (9.7309, -64.8547) (9.7759, -64.9327) (9.8212, -65.0106) (9.8669, -65.0884) (9.9129, -65.166) (9.9592, -65.2436) (10.0058, -65.321) (10.0527, -65.3984) (10.0999, -65.4756) (10.1475, -65.5527) (10.1954, -65.6298) (10.2435, -65.7067) (10.292, -65.7835) (10.3408, -65.8602) (10.3898, -65.9368) (10.4392, -66.0133) (10.4789, -66.0744) (10.5089, -66.1202) (10.5289, -66.1507) (10.5389, -66.1659) knots 0.270845 0.270845 0.270845 0.270845 0.270845 0.270845 0.271429 0.285714 0.3 0.314286 0.328571 0.342857 0.357143 0.371429 0.385714 0.4 0.414286 0.428571 0.442857 0.457143 0.471429 0.485714 0.5 0.514286 0.528571 0.542857 0.557143 0.571429 0.585714 0.6 0.614286 0.628571 0.642857 0.657143 0.671429 0.685714 0.7 0.714286 0.728571 0.742857 0.757143 0.771429 0.785714 0.8 0.814286 0.828571 0.842857 0.857143 0.871429 0.885714 0.9 0.914286 0.928571 0.942857 0.957143 0.971429 0.985714 1 1 1 1 1 1
  arc A37 (10.5389, -66.1659) -> (12.0195, -65.9131) centre (0, 0) ccw
  spline S74 degree 5 poles (12.0195, -65.9131) (12.0239, -65.8954) (12.0327, -65.8599) (12.0457, -65.8068) (12.0629, -65.736) (12.0841, -65.6474) (12.1049, -65.5589) (12.1255, -65.4703) (12.1457, -65.3818) (12.1656, -65.2933) (12.1852, -65.2047) (12.2045, -65.1162) (12.2234, -65.0276) (12.242, -64.9391) (12.2603, -64.8506) (12.2782, -64.762) (12.2958, -64.6735) (12.3131, -64.585) (12.33, -64.4965) (12.3466, -64.408) (12.3628, -64.3195) (12.3787, -64.231) (12.3942, -64.1426) (12.4093, -64.0541) (12.4242, -63.9657) (12.4386, -63.8772) (12.4527, -63.7888) (12.4664, -63.7004) (12.4798, -63.612) (12.4927, -63.5237) (12.5053, -63.4353) (12.5175, -63.347) (12.5294, -63.2587) (12.5408, -63.1704) (12.5519, -63.0822) (12.5625, -62.9939) (12.5727, -62.9057) (12.5826, -62.8175) (12.592, -62.7294) (12.601, -62.6413) (12.6096, -62.5532) (12.6177, -62.4651) (12.6255, -62.3771) (12.6327, -62.2891) (12.6396, -62.2012) (12.646, -62.1133) (12.6519, -62.0254) (12.6573, -61.9376) (12.6623, -61.8499) (12.6667, -61.7622) (12.6707, -61.6745) (12.6742, -61.5869) (12.6766, -61.5161) (12.6782, -61.4629) (12.6791, -61.4272) (12.6796, -61.409) (12.6796, -61.4083) knots -1 -1 -1 -1 -1 -1 -0.985714 -0.971429 -0.957143 -0.942857 -0.928571 -0.914286 -0.9 -0.885714 -0.871429 -0.857143 -0.842857 -0.828571 -0.814286 -0.8 -0.785714 -0.771429 -0.757143 -0.742857 -0.728571 -0.714286 -0.7 -0.685714 -0.671429 -0.657143 -0.642857 -0.628571 -0.614286 -0.6 -0.585714 -0.571429 -0.557143 -0.542857 -0.528571 -0.514286 -0.5 -0.485714 -0.471429 -0.457143 -0.442857 -0.428571 -0.414286 -0.4 -0.385714 -0.371429 -0.357143 -0.342857 -0.328571 -0.314286 -0.3 -0.285714 -0.271429 -0.270845 -0.270845 -0.270845 -0.270845 -0.270845 -0.270845
  spline S75 degree 3 poles (12.8385, -61.2175) (12.813, -61.2228) (12.7888, -61.2331) (12.7457, -61.2623) (12.7272, -61.281) (12.7025, -61.3183) (12.6944, -61.3353) (12.6831, -61.371) (12.68, -61.3895) (12.6796, -61.4083) knots 0 0 0 0 0.007813 0.007813 0.015626 0.015626 0.021241 0.021241 0.026855 0.026855 0.026855 0.026855
  arc A38 (12.8385, -61.2175) -> (14.1542, -60.9267) centre (0, 0) ccw
  spline S76 degree 3 poles (14.3787, -61.0328) (14.3672, -61.0094) (14.3512, -60.9886) (14.3121, -60.9542) (14.2893, -60.9409) (14.247, -60.9263) (14.2286, -60.9227) (14.1912, -60.9208) (14.1725, -60.9224) (14.1542, -60.9267) knots 0 0 0 0 0.007813 0.007813 0.015626 0.015626 0.021241 0.021241 0.026855 0.026855 0.026855 0.026855
  spline S77 degree 5 poles (14.3787, -61.0328) (14.379, -61.0334) (14.3871, -61.0497) (14.403, -61.0817) (14.4269, -61.1293) (14.4589, -61.1925) (14.4989, -61.2705) (14.5395, -61.3483) (14.5805, -61.426) (14.622, -61.5035) (14.6639, -61.5808) (14.7063, -61.658) (14.7491, -61.735) (14.7924, -61.8119) (14.8361, -61.8886) (14.8802, -61.9652) (14.9247, -62.0416) (14.9696, -62.1178) (15.0149, -62.194) (15.0606, -62.2699) (15.1066, -62.3458) (15.1531, -62.4214) (15.1999, -62.497) (15.2471, -62.5723) (15.2947, -62.6476) (15.3427, -62.7227) (15.3909, -62.7976) (15.4396, -62.8724) (15.4886, -62.9471) (15.5379, -63.0216) (15.5876, -63.096) (15.6377, -63.1703) (15.688, -63.2444) (15.7387, -63.3183) (15.7898, -63.3922) (15.8411, -63.4658) (15.8928, -63.5394) (15.9448, -63.6128) (15.9972, -63.6861) (16.0498, -63.7592) (16.1027, -63.8322) (16.156, -63.9051) (16.2096, -63.9778) (16.2634, -64.0504) (16.3176, -64.1228) (16.3721, -64.1952) (16.4269, -64.2673) (16.482, -64.3394) (16.5373, -64.4113) (16.593, -64.4831) (16.6489, -64.5547) (16.7052, -64.6262) (16.7617, -64.6976) (16.8071, -64.7546) (16.8413, -64.7973) (16.8642, -64.8257) (16.8756, -64.8399) knots 0.270845 0.270845 0.270845 0.270845 0.270845 0.270845 0.271429 0.285714 0.3 0.314286 0.328571 0.342857 0.357143 0.371429 0.385714 0.4 0.414286 0.428571 0.442857 0.457143 0.471429 0.485714 0.5 0.514286 0.528571 0.542857 0.557143 0.571429 0.585714 0.6 0.614286 0.628571 0.642857 0.657143 0.671429 0.685714 0.7 0.714286 0.728571 0.742857 0.757143 0.771429 0.785714 0.8 0.814286 0.828571 0.842857 0.857143 0.871429 0.885714 0.9 0.914286 0.928571 0.942857 0.957143 0.971429 0.985714 1 1 1 1 1 1
  arc A39 (16.8756, -64.8399) -> (18.3249, -64.4453) centre (0, 0) ccw
  spline S78 degree 5 poles (18.3249, -64.4453) (18.3276, -64.4273) (18.3329, -64.3912) (18.3407, -64.337) (18.351, -64.2649) (18.3636, -64.1747) (18.3758, -64.0845) (18.3877, -63.9944) (18.3993, -63.9043) (18.4105, -63.8143) (18.4215, -63.7243) (18.4321, -63.6343) (18.4424, -63.5443) (18.4524, -63.4544) (18.462, -63.3645) (18.4713, -63.2747) (18.4803, -63.1849) (18.4889, -63.0951) (18.4972, -63.0054) (18.5052, -62.9157) (18.5128, -62.8261) (18.5201, -62.7365) (18.527, -62.6469) (18.5335, -62.5574) (18.5397, -62.4679) (18.5456, -62.3785) (18.5511, -62.2892) (18.5562, -62.1998) (18.5609, -62.1106) (18.5653, -62.0214) (18.5693, -61.9322) (18.573, -61.8431) (18.5762, -61.7541) (18.5791, -61.6651) (18.5816, -61.5762) (18.5836, -61.4874) (18.5853, -61.3986) (18.5866, -61.3099) (18.5875, -61.2212) (18.5879, -61.1327) (18.588, -61.0442) (18.5876, -60.9557) (18.5868, -60.8674) (18.5855, -60.7791) (18.5839, -60.6909) (18.5817, -60.6028) (18.5791, -60.5148) (18.5761, -60.4269) (18.5725, -60.339) (18.5685, -60.2513) (18.564, -60.1637) (18.559, -60.0761) (18.5546, -60.0055) (18.551, -59.9523) (18.5485, -59.9167) (18.5472, -59.8985) (18.5471, -59.8978) knots -1 -1 -1 -1 -1 -1 -0.985714 -0.971429 -0.957143 -0.942857 -0.928571 -0.914286 -0.9 -0.885714 -0.871429 -0.857143 -0.842857 -0.828571 -0.814286 -0.8 -0.785714 -0.771429 -0.757143 -0.742857 -0.728571 -0.714286 -0.7 -0.685714 -0.671429 -0.657143 -0.642857 -0.628571 -0.614286 -0.6 -0.585714 -0.571429 -0.557143 -0.542857 -0.528571 -0.514286 -0.5 -0.485714 -0.471429 -0.457143 -0.442857 -0.428571 -0.414286 -0.4 -0.385714 -0.371429 -0.357143 -0.342857 -0.328571 -0.314286 -0.3 -0.285714 -0.271429 -0.270845 -0.270845 -0.270845 -0.270845 -0.270845 -0.270845
  spline S79 degree 3 poles (18.6869, -59.6926) (18.662, -59.7004) (18.6389, -59.7129) (18.5988, -59.7462) (18.5822, -59.7666) (18.5612, -59.8061) (18.5548, -59.8238) (18.5471, -59.8604) (18.5458, -59.8792) (18.5471, -59.8978) knots 0 0 0 0 0.007813 0.007813 0.015626 0.015626 0.021241 0.021241 0.026855 0.026855 0.026855 0.026855
  arc A40 (18.6869, -59.6926) -> (19.9684, -59.2762) centre (0, 0) ccw
  spline S80 degree 3 poles (20.2021, -59.3601) (20.1884, -59.338) (20.1704, -59.3188) (20.1282, -59.2883) (20.1043, -59.2773) (20.0608, -59.2669) (20.042, -59.2651) (20.0046, -59.2667) (19.9862, -59.2702) (19.9684, -59.2762) knots 0 0 0 0 0.007813 0.007813 0.015626 0.015626 0.021241 0.021241 0.026855 0.026855 0.026855 0.026855
  spline S81 degree 5 poles (20.2021, -59.3601) (20.2025, -59.3607) (20.2121, -59.3762) (20.231, -59.4065) (20.2594, -59.4516) (20.2973, -59.5113) (20.3447, -59.5851) (20.3926, -59.6586) (20.4409, -59.732) (20.4897, -59.8051) (20.5389, -59.878) (20.5885, -59.9508) (20.6386, -60.0233) (20.6891, -60.0957) (20.7399, -60.1678) (20.7912, -60.2397) (20.8429, -60.3115) (20.8949, -60.3831) (20.9474, -60.4545) (21.0002, -60.5257) (21.0533, -60.5967) (21.1069, -60.6675) (21.1608, -60.7382) (21.2151, -60.8087) (21.2697, -60.879) (21.3246, -60.9491) (21.3799, -61.019) (21.4356, -61.0888) (21.4916, -61.1584) (21.5479, -61.2278) (21.6045, -61.297) (21.6615, -61.3661) (21.7188, -61.435) (21.7764, -61.5037) (21.8343, -61.5723) (21.8925, -61.6407) (21.9511, -61.7089) (22.0099, -61.7769) (22.0691, -61.8448) (22.1285, -61.9125) (22.1883, -61.9801) (22.2483, -62.0475) (22.3086, -62.1147) (22.3693, -62.1817) (22.4302, -62.2486) (22.4914, -62.3153) (22.5529, -62.3819) (22.6147, -62.4483) (22.6767, -62.5145) (22.739, -62.5806) (22.8016, -62.6465) (22.8645, -62.7122) (22.9277, -62.7778) (22.9784, -62.8302) (23.0166, -62.8693) (23.0421, -62.8954) (23.0548, -62.9085) knots 0.270845 0.270845 0.270845 0.270845 0.270845 0.270845 0.271429 0.285714 0.3 0.314286 0.328571 0.342857 0.357143 0.371429 0.385714 0.4 0.414286 0.428571 0.442857 0.457143 0.471429 0.485714 0.5 0.514286 0.528571 0.542857 0.557143 0.571429 0.585714 0.6 0.614286 0.628571 0.642857 0.657143 0.671429 0.685714 0.7 0.714286 0.728571 0.742857 0.757143 0.771429 0.785714 0.8 0.814286 0.828571 0.842857 0.857143 0.871429 0.885714 0.9 0.914286 0.928571 0.942857 0.957143 0.971429 0.985714 1 1 1 1 1 1
  arc A41 (23.0548, -62.9085) -> (24.4592, -62.3758) centre (0, 0) ccw
  spline S82 degree 5 poles (24.4592, -62.3758) (24.4602, -62.3576) (24.4619, -62.3212) (24.4645, -62.2665) (24.4678, -62.1937) (24.4716, -62.1028) (24.475, -62.0119) (24.4782, -61.921) (24.481, -61.8302) (24.4836, -61.7395) (24.4858, -61.6489) (24.4877, -61.5583) (24.4892, -61.4677) (24.4905, -61.3773) (24.4914, -61.2869) (24.492, -61.1966) (24.4922, -61.1063) (24.4922, -61.0161) (24.4918, -60.926) (24.491, -60.836) (24.49, -60.746) (24.4885, -60.6561) (24.4868, -60.5663) (24.4847, -60.4766) (24.4822, -60.387) (24.4794, -60.2974) (24.4762, -60.2079) (24.4727, -60.1185) (24.4688, -60.0292) (24.4646, -59.94) (24.46, -59.8509) (24.455, -59.7619) (24.4496, -59.673) (24.4439, -59.5841) (24.4378, -59.4954) (24.4313, -59.4068) (24.4244, -59.3182) (24.4171, -59.2298) (24.4094, -59.1415) (24.4013, -59.0533) (24.3928, -58.9652) (24.3839, -58.8772) (24.3746, -58.7894) (24.3648, -58.7016) (24.3546, -58.614) (24.344, -58.5265) (24.3329, -58.4392) (24.3214, -58.3519) (24.3094, -58.2649) (24.2969, -58.1779) (24.284, -58.0911) (24.2706, -58.0045) (24.2593, -57.9346) (24.2506, -57.882) (24.2447, -57.8468) (24.2416, -57.8288) (24.2415, -57.8281) knots -1 -1 -1 -1 -1 -1 -0.985714 -0.971429 -0.957143 -0.942857 -0.928571 -0.914286 -0.9 -0.885714 -0.871429 -0.857143 -0.842857 -0.828571 -0.814286 -0.8 -0.785714 -0.771429 -0.757143 -0.742857 -0.728571 -0.714286 -0.7 -0.685714 -0.671429 -0.657143 -0.642857 -0.628571 -0.614286 -0.6 -0.585714 -0.571429 -0.557143 -0.542857 -0.528571 -0.514286 -0.5 -0.485714 -0.471429 -0.457143 -0.442857 -0.428571 -0.414286 -0.4 -0.385714 -0.371429 -0.357143 -0.342857 -0.328571 -0.314286 -0.3 -0.285714 -0.271429 -0.270845 -0.270845 -0.270845 -0.270845 -0.270845 -0.270845
  spline S83 degree 3 poles (24.3608, -57.6104) (24.3368, -57.6205) (24.315, -57.6352) (24.2784, -57.6722) (24.2638, -57.6941) (24.2467, -57.7355) (24.242, -57.7537) (24.2378, -57.7909) (24.2384, -57.8097) (24.2415, -57.8281) knots 0 0 0 0 0.007813 0.007813 0.015626 0.015626 0.021241 0.021241 0.026855 0.026855 0.026855 0.026855
  arc A42 (24.3608, -57.6104) -> (25.5962, -57.0722) centre (0, 0) ccw
  spline S84 degree 3 poles (25.8369, -57.1332) (25.8211, -57.1125) (25.8013, -57.0951) (25.7564, -57.0689) (25.7315, -57.0602) (25.6872, -57.054) (25.6684, -57.0541) (25.6313, -57.0593) (25.6133, -57.0646) (25.5962, -57.0722) knots 0 0 0 0 0.007813 0.007813 0.015626 0.015626 0.021241 0.021241 0.026855 0.026855 0.026855 0.026855
  spline S85 degree 5 poles (25.8369, -57.1332) (25.8373, -57.1338) (25.8484, -57.1482) (25.8701, -57.1766) (25.9027, -57.2187) (25.9462, -57.2745) (26.0005, -57.3434) (26.0553, -57.412) (26.1105, -57.4803) (26.166, -57.5484) (26.2221, -57.6162) (26.2785, -57.6838) (26.3353, -57.7512) (26.3925, -57.8183) (26.4501, -57.8852) (26.5081, -57.9519) (26.5665, -58.0183) (26.6252, -58.0845) (26.6843, -58.1505) (26.7437, -58.2163) (26.8035, -58.2819) (26.8636, -58.3472) (26.9241, -58.4123) (26.9849, -58.4772) (27.046, -58.5419) (27.1075, -58.6064) (27.1693, -58.6707) (27.2314, -58.7348) (27.2939, -58.7986) (27.3566, -58.8623) (27.4197, -58.9257) (27.483, -58.989) (27.5467, -59.052) (27.6107, -59.1149) (27.6749, -59.1775) (27.7395, -59.24) (27.8044, -59.3022) (27.8695, -59.3643) (27.9349, -59.4261) (28.0006, -59.4878) (28.0666, -59.5493) (28.1329, -59.6105) (28.1994, -59.6716) (28.2663, -59.7325) (28.3333, -59.7932) (28.4007, -59.8537) (28.4683, -59.914) (28.5362, -59.9741) (28.6044, -60.0341) (28.6728, -60.0938) (28.7414, -60.1534) (28.8104, -60.2127) (28.8796, -60.2719) (28.9351, -60.3191) (28.9769, -60.3544) (29.0048, -60.3779) (29.0187, -60.3897) knots 0.270845 0.270845 0.270845 0.270845 0.270845 0.270845 0.271429 0.285714 0.3 0.314286 0.328571 0.342857 0.357143 0.371429 0.385714 0.4 0.414286 0.428571 0.442857 0.457143 0.471429 0.485714 0.5 0.514286 0.528571 0.542857 0.557143 0.571429 0.585714 0.6 0.614286 0.628571 0.642857 0.657143 0.671429 0.685714 0.7 0.714286 0.728571 0.742857 0.757143 0.771429 0.785714 0.8 0.814286 0.828571 0.842857 0.857143 0.871429 0.885714 0.9 0.914286 0.928571 0.942857 0.957143 0.971429 0.985714 1 1 1 1 1 1
  arc A43 (29.0187, -60.3897) -> (30.3652, -59.724) centre (0, 0) ccw
  spline S86 degree 5 poles (30.3652, -59.724) (30.3643, -59.7058) (30.3626, -59.6693) (30.3599, -59.6147) (30.3561, -59.5419) (30.3511, -59.451) (30.3458, -59.3602) (30.3402, -59.2695) (30.3342, -59.1788) (30.328, -59.0883) (30.3214, -58.9978) (30.3146, -58.9075) (30.3074, -58.8172) (30.2999, -58.7271) (30.2921, -58.637) (30.284, -58.547) (30.2755, -58.4572) (30.2667, -58.3674) (30.2576, -58.2778) (30.2482, -58.1882) (30.2385, -58.0988) (30.2284, -58.0095) (30.218, -57.9203) (30.2072, -57.8312) (30.1961, -57.7422) (30.1847, -57.6533) (30.1729, -57.5646) (30.1607, -57.4759) (30.1483, -57.3874) (30.1354, -57.299) (30.1222, -57.2108) (30.1087, -57.1227) (30.0948, -57.0347) (30.0805, -56.9468) (30.0658, -56.8591) (30.0508, -56.7715) (30.0354, -56.684) (30.0196, -56.5967) (30.0034, -56.5096) (29.9869, -56.4225) (29.9699, -56.3357) (29.9525, -56.249) (29.9348, -56.1624) (29.9166, -56.076) (29.898, -55.9898) (29.879, -55.9038) (29.8595, -55.8179) (29.8396, -55.7322) (29.8193, -55.6467) (29.7985, -55.5613) (29.7772, -55.4762) (29.7555, -55.3912) (29.7376, -55.3227) (29.7238, -55.2713) (29.7145, -55.2368) (29.7098, -55.2192) (29.7096, -55.2185) knots -1 -1 -1 -1 -1 -1 -0.985714 -0.971429 -0.957143 -0.942857 -0.928571 -0.914286 -0.9 -0.885714 -0.871429 -0.857143 -0.842857 -0.828571 -0.814286 -0.8 -0.785714 -0.771429 -0.757143 -0.742857 -0.728571 -0.714286 -0.7 -0.685714 -0.671429 -0.657143 -0.642857 -0.628571 -0.614286 -0.6 -0.585714 -0.571429 -0.557143 -0.542857 -0.528571 -0.514286 -0.5 -0.485714 -0.471429 -0.457143 -0.442857 -0.428571 -0.414286 -0.4 -0.385714 -0.371429 -0.357143 -0.342857 -0.328571 -0.314286 -0.3 -0.285714 -0.271429 -0.270845 -0.270845 -0.270845 -0.270845 -0.270845 -0.270845
  spline S87 degree 3 poles (29.8073, -54.9903) (29.7844, -55.0027) (29.7641, -55.0194) (29.7312, -55.0598) (29.7188, -55.083) (29.7058, -55.1258) (29.7029, -55.1444) (29.7023, -55.1818) (29.7047, -55.2005) (29.7096, -55.2185) knots 0 0 0 0 0.007813 0.007813 0.015626 0.015626 0.021241 0.021241 0.026855 0.026855 0.026855 0.026855
  arc A44 (29.8073, -54.9903) -> (30.9849, -54.3354) centre (0, 0) ccw
  spline S88 degree 3 poles (31.2304, -54.3729) (31.2127, -54.3538) (31.1914, -54.3384) (31.1441, -54.3166) (31.1185, -54.3104) (31.0738, -54.3085) (31.0551, -54.3104) (31.0187, -54.3192) (31.0012, -54.3261) (30.9849, -54.3354) knots 0 0 0 0 0.007813 0.007813 0.015626 0.015626 0.021241 0.021241 0.026855 0.026855 0.026855 0.026855
  spline S89 degree 5 poles (31.2304, -54.3729) (31.2309, -54.3734) (31.2433, -54.3867) (31.2677, -54.4128) (31.3042, -54.4516) (31.3529, -54.503) (31.4136, -54.5663) (31.4747, -54.6292) (31.5362, -54.6919) (31.5981, -54.7543) (31.6604, -54.8165) (31.7231, -54.8783) (31.7862, -54.9399) (31.8496, -55.0012) (31.9134, -55.0622) (31.9775, -55.1229) (32.042, -55.1834) (32.1069, -55.2437) (32.172, -55.3037) (32.2375, -55.3634) (32.3034, -55.4229) (32.3695, -55.4821) (32.436, -55.5411) (32.5028, -55.5998) (32.5699, -55.6583) (32.6373, -55.7166) (32.705, -55.7746) (32.773, -55.8324) (32.8413, -55.8899) (32.9099, -55.9472) (32.9788, -56.0043) (33.048, -56.0611) (33.1175, -56.1177) (33.1872, -56.1741) (33.2572, -56.2302) (33.3275, -56.2862) (33.398, -56.3419) (33.4689, -56.3973) (33.54, -56.4526) (33.6113, -56.5076) (33.6829, -56.5624) (33.7548, -56.617) (33.8269, -56.6714) (33.8993, -56.7256) (33.9719, -56.7795) (34.0448, -56.8332) (34.118, -56.8867) (34.1913, -56.94) (34.265, -56.9931) (34.3388, -57.0459) (34.4129, -57.0986) (34.4872, -57.151) (34.5618, -57.2033) (34.6217, -57.2449) (34.6666, -57.276) (34.6967, -57.2967) (34.7117, -57.307) knots 0.270845 0.270845 0.270845 0.270845 0.270845 0.270845 0.271429 0.285714 0.3 0.314286 0.328571 0.342857 0.357143 0.371429 0.385714 0.4 0.414286 0.428571 0.442857 0.457143 0.471429 0.485714 0.5 0.514286 0.528571 0.542857 0.557143 0.571429 0.585714 0.6 0.614286 0.628571 0.642857 0.657143 0.671429 0.685714 0.7 0.714286 0.728571 0.742857 0.757143 0.771429 0.785714 0.8 0.814286 0.828571 0.842857 0.857143 0.871429 0.885714 0.9 0.914286 0.928571 0.942857 0.957143 0.971429 0.985714 1 1 1 1 1 1
  arc A45 (34.7117, -57.307) -> (35.9876, -56.5145) centre (0, 0) ccw
  spline S90 degree 5 poles (35.9876, -56.5145) (35.985, -56.4965) (35.9798, -56.4603) (35.9718, -56.4062) (35.961, -56.3341) (35.9473, -56.2441) (35.9332, -56.1543) (35.9189, -56.0645) (35.9042, -55.9749) (35.8892, -55.8854) (35.874, -55.796) (35.8584, -55.7067) (35.8426, -55.6176) (35.8264, -55.5285) (35.81, -55.4397) (35.7932, -55.3509) (35.7761, -55.2623) (35.7587, -55.1738) (35.741, -55.0854) (35.723, -54.9972) (35.7046, -54.9092) (35.686, -54.8212) (35.667, -54.7334) (35.6477, -54.6458) (35.6281, -54.5583) (35.6081, -54.4709) (35.5878, -54.3837) (35.5672, -54.2967) (35.5462, -54.2098) (35.5249, -54.1231) (35.5033, -54.0365) (35.4813, -53.9501) (35.4589, -53.8638) (35.4362, -53.7778) (35.4132, -53.6919) (35.3898, -53.6061) (35.366, -53.5206) (35.3418, -53.4352) (35.3173, -53.35) (35.2924, -53.265) (35.2672, -53.1802) (35.2415, -53.0955) (35.2155, -53.0111) (35.189, -52.9269) (35.1622, -52.8429) (35.135, -52.759) (35.1073, -52.6754) (35.0792, -52.5921) (35.0507, -52.5089) (35.0218, -52.426) (34.9924, -52.3433) (34.9626, -52.2608) (34.9382, -52.1944) (34.9195, -52.1445) (34.9069, -52.1111) (34.9005, -52.094) (34.9002, -52.0934) knots -1 -1 -1 -1 -1 -1 -0.985714 -0.971429 -0.957143 -0.942857 -0.928571 -0.914286 -0.9 -0.885714 -0.871429 -0.857143 -0.842857 -0.828571 -0.814286 -0.8 -0.785714 -0.771429 -0.757143 -0.742857 -0.728571 -0.714286 -0.7 -0.685714 -0.671429 -0.657143 -0.642857 -0.628571 -0.614286 -0.6 -0.585714 -0.571429 -0.557143 -0.542857 -0.528571 -0.514286 -0.5 -0.485714 -0.471429 -0.457143 -0.442857 -0.428571 -0.414286 -0.4 -0.385714 -0.371429 -0.357143 -0.342857 -0.328571 -0.314286 -0.3 -0.285714 -0.271429 -0.270845 -0.270845 -0.270845 -0.270845 -0.270845 -0.270845
  spline S91 degree 3 poles (34.9754, -51.8567) (34.9539, -51.8713) (34.9353, -51.8899) (34.9064, -51.9333) (34.8963, -51.9576) (34.8875, -52.0014) (34.8864, -52.0202) (34.8895, -52.0575) (34.8936, -52.0759) (34.9002, -52.0934) knots 0 0 0 0 0.007813 0.007813 0.015626 0.015626 0.021241 0.021241 0.026855 0.026855 0.026855 0.026855
  arc A46 (34.9754, -51.8567) -> (36.0844, -51.0913) centre (0, 0) ccw
  spline S92 degree 3 poles (36.3323, -51.1049) (36.3128, -51.0876) (36.2902, -51.0743) (36.241, -51.0572) (36.2149, -51.0535) (36.1702, -51.0559) (36.1518, -51.0596) (36.1164, -51.0719) (36.0997, -51.0805) (36.0844, -51.0913) knots 0 0 0 0 0.007813 0.007813 0.015626 0.015626 0.021241 0.021241 0.026855 0.026855 0.026855 0.026855